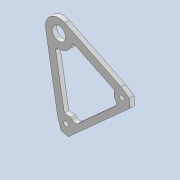
# Autodesk Inventor part: stand_3
Saved by Autodesk Inventor 2020 (Build 240168000, 168)
## iProperties
Created: 2021-07-20
Part Number: stand_3
Material: Generic
Document SubType Name: Modeling
Designer: Shuang Peng
Density: 1 g/cm^3
Appearance: Default
Author: Shuang Peng
Autodesk Inventor part; units mm, degrees
ref_plane "YZ Plane" through (0, 0, 0) normal (1, 0, 0) x (0, 1, 0)
ref_plane "XZ Plane" through (0, 0, 0) normal (0, 1, 0) x (-1, 0, 0)
ref_plane "XY Plane" through (0, 0, 0) normal (0, 0, 1) x (1, 0, 0)
sketch "Sketch1" plane through (0, 0, 0) normal (0, 0, 1) x (1, 0, 0)
  circle A0 centre (10.538, 13.901) radius 1.5 projected
  circle A1 centre (-14.3574, -8.5148) radius 1.5 projected
  line L0 (-15.1125, -4.8626) -> (-12.2879, -5.0107) projected
  line L1 (-15.1125, -4.8626) -> (-18.0851, -7.5392) projected
  line L2 (-15.5871, -15.1392) -> (-18.0851, -7.5392) projected
  line L3 (16.4403, 13.6984) -> (-15.5871, -15.1392) projected
  line L4 (16.4403, 13.6984) -> (10.1865, 17.9166) projected
  line L5 (10.1865, 17.9166) -> (7.2139, 15.2401) projected
  line L6 (7.0659, 12.4156) -> (7.2139, 15.2401) projected
  line L7 (7.0659, 12.4156) -> (7.6141, 11.8066) projected
  arc A2 (7.4661, 8.9821) -> (7.6141, 11.8066) centre (6.1278, 10.4684) ccw projected
  line L8 (-8.9151, -5.7676) -> (7.4661, 8.9821) projected
  arc A3 (-11.7396, -5.6196) -> (-8.9151, -5.7676) centre (-10.2534, -4.2813) ccw projected
  line L9 (-11.7396, -5.6196) -> (-12.2879, -5.0107) projected
  circle A4 centre (-17.5227, 24.7135) radius 1.5 projected
  circle A5 centre (-17.5227, 24.7135) radius 3
  circle A6 centre (-17.5227, 24.7135) radius 6
  line L10 (-18.0851, -7.5392) -> (-23.4365, 23.7005)
  line L11 (10.1865, 17.9166) -> (-14.8998, 30.1099)
  line L12 (-15.1125, -4.8626) -> (-19.1917, 18.9503)
  line L13 (7.2139, 15.2401) -> (-11.5335, 24.3523)
  point P0 (0, 0)
  dimension "d0" = 6
  dimension "d1" = 12
  constraints: 8 end point, 4 point on circle, 2 centre point, 2 coincident, 2 parallel, 2 tangent
  measures "d0" diameter of A5
  measures "d1" diameter of A6
extrude "Extrusion1" add sketch "Sketch1" along normal blind 2 contours L0 L9 A3 L8 A2 L7 L6 L5 L4 L3 L2 L1 | L1 L10 A6 L12 | A6 | A6 L11 L5 L13
chamfer "Chamfer1" distance 3 angle 45 2 edges at (16.4403, 13.6984, 1) (-15.5871, -15.1392, 1)
sketch "Sketch2" plane through (0, 0, 2) normal (0, 0, 1) x (1, 0, 0)
  line L0 (-13.3576, -13.1318) -> (-16.5238, -12.2892) projected
  line L1 (-13.3576, -13.1318) -> (14.2108, 11.691) projected
  line L2 (13.9532, 15.376) -> (14.2108, 11.691) projected
  line L3 (13.9532, 15.376) -> (10.1865, 17.9166) projected
  line L4 (10.1865, 17.9166) -> (-14.8998, 30.1099) projected
  arc A0 (-14.8998, 30.1099) -> (-23.4365, 23.7005) centre (-17.5227, 24.7135) ccw projected
  line L5 (-23.4365, 23.7005) -> (-18.0851, -7.5392) projected
  line L6 (-18.0851, -7.5392) -> (-16.5238, -12.2892) projected
  circle A1 centre (-17.5227, 24.7135) radius 3 projected
  circle A2 centre (10.538, 13.901) radius 1.5 projected
  circle A3 centre (-14.3574, -8.5148) radius 1.5 projected
  line L7 (-15.1125, -4.8626) -> (-19.1917, 18.9503) projected
  arc A4 (-19.1917, 18.9503) -> (-11.5335, 24.3523) centre (-17.5227, 24.7135) ccw projected
  line L8 (-11.5335, 24.3523) -> (7.2139, 15.2401) projected
  line L9 (7.2139, 15.2401) -> (7.0659, 12.4156) projected
  line L10 (7.0659, 12.4156) -> (7.6141, 11.8066) projected
  arc A5 (7.4661, 8.9821) -> (7.6141, 11.8066) centre (6.1278, 10.4684) ccw projected
  line L11 (7.4661, 8.9821) -> (-8.9151, -5.7676) projected
  arc A6 (-11.7396, -5.6196) -> (-8.9151, -5.7676) centre (-10.2534, -4.2813) ccw projected
  line L12 (-11.7396, -5.6196) -> (-12.2879, -5.0107) projected
  line L13 (-12.2879, -5.0107) -> (-15.1125, -4.8626) projected
  circle A7 centre (-14.3574, -8.5148) radius 1.5 projected
  circle A8 centre (-14.3574, -8.5148) radius 1
  circle A9 centre (10.538, 13.901) radius 1
  point P0 (0, 0)
  dimension "d7" = 2
  dimension "d8" = 2
  constraints: 2 centre point, 2 coincident
  measures "d7" diameter of A8
  measures "d8" diameter of A9
extrude "Extrusion2" add sketch "Sketch2" against normal blind 2 contours A2 | A3
fillet "Fillet1" radius 1 2 edges at (-19.1917, 18.9503, 1) (-11.5335, 24.3523, 1)
body "Solid1"
